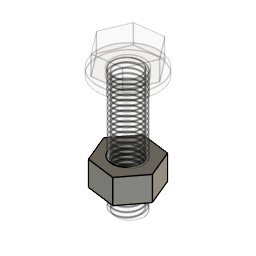
M10_Assembly_Final (Autodesk Fusion 360 design; units mm, degrees)
part number: 2026-04-25-14-00-48-438
part number: 2026-04-25-14-02-05-516
part number: 2026-04-25-14-04-24-538
part number: 2026-04-25-14-13-24-813
Autodesk Fusion 360 part; units mm, degrees
sketch "Sketch1" plane through (0, 0, 0) normal (0, 0, 1) x (1, 0, 0) in component "Washer"
  circle A0 centre (0, 0) radius 10
  circle A1 centre (0, 0) radius 5.25
  dimension "d1" = 20
  dimension "d2" = 10.5
  constraint coincident A0.centre A1.centre
  constraint concentric A0 A1
  measures "d1" diameter of A0
  measures "d2" diameter of A1
extrude "Extrude1" add sketch "Sketch1" along normal blind 2 makes body 1 in component "Washer"
sketch "Sketch1 (2)" plane through (0, 0, 2) normal (0, 0, 1) x (-1, 0, 0) in component "Bolt"
  circle A0 centre (0, 0) radius 5.25
  circle A1 centre (0, 0) radius 10
  line L0 (-3.5698, -8.5199) -> (5.5936, -7.3516)
  line L1 (5.5936, -7.3516) -> (9.1634, 1.1684)
  line L2 (9.1634, 1.1684) -> (3.5698, 8.5199)
  line L3 (3.5698, 8.5199) -> (-5.5936, 7.3516)
  line L4 (-5.5936, 7.3516) -> (-9.1634, -1.1684)
  line L5 (-9.1634, -1.1684) -> (-3.5698, -8.5199)
  dimension "d5" = 8
  constraint coincident A0.centre A1.centre
  measures "d5" distance of A0.centre L5
extrude "Extrude1'" add sketch "Sketch1 (2)" along normal blind 6.4 separate body contours A0 | L0 L1 L2 L3 L4 L5 makes body 2 in component "Bolt"
sketch "Sketch2" plane through (0, 0, 2) normal (0, 0, -1) x (1, 0, 0) in component "Bolt"
  line L0 (3.5698, -8.5199) -> (9.1634, -1.1684)
  line L1 (9.1634, -1.1684) -> (5.5936, 7.3516)
  line L2 (5.5936, 7.3516) -> (-3.5698, 8.5199)
  line L3 (-3.5698, 8.5199) -> (-9.1634, 1.1684)
  line L4 (-9.1634, 1.1684) -> (-5.5936, -7.3516)
  line L5 (-5.5936, -7.3516) -> (3.5698, -8.5199)
  circle A0 centre (0, 0) radius 5
  dimension "d8" = 10
  constraint coincident A0.centre origin
  measures "d8" diameter of A0
extrude "Extrude2" add sketch "Sketch2" along normal blind 40 contours A0 bodies 2 in component "Bolt"
thread "Thread1" "ISO Metric profile 10.0 M10x1.5 M10x1.5 6g" major diameter 9.85 minor diameter 8.141 pitch 1.5 angle 60 modelled right hand crest width 0.2177 on face at (4.9938, 0.2492, -24.6667) crest through (4.925, 0, 2.375) on bodies 2 in component "Bolt"
sketch "Sketch1 (3)" plane through (0, 0, -38) normal (0, 0, -1) x (1, 0, 0) in component "Nut"
  spline S0 degree 3 poles (-4.0519, -0.3884) (-4.055, -0.9258) (-3.9512, -1.4584) (-3.5409, -2.4749) (-3.2312, -2.9459) (-2.4367, -3.7605) (-1.9541, -4.0907) (-0.8716, -4.5594) (-0.2791, -4.6862) (0.7385, -4.7058) (1.1549, -4.6582) (1.9739, -4.4542) (2.3723, -4.2963) (2.7453, -4.0889) knots 0 0 0 0 0.161221 0.161221 0.328565 0.328565 0.502029 0.502029 0.68161 0.68161 0.806401 0.806401 0.933976 0.933976 0.933976 0.933976
  arc A0 (2.7453, -4.0889) -> (4.9137, -0.3331) centre (0, 0) ccw
  spline S1 degree 3 poles (4.9137, -0.3331) (4.9036, 0.2959) (4.7727, 0.9169) (4.2847, 2.0534) (3.9396, 2.5608) (3.0865, 3.3975) (2.5922, 3.7244) (1.5238, 4.1587) (0.9631, 4.2693) (0.0275, 4.2662) (-0.3405, 4.2169) (-1.0448, 4.0248) (-1.3786, 3.8852) (-1.6896, 3.7033) knots 0 0 0 0 0.188714 0.188714 0.371292 0.371292 0.547732 0.547732 0.718032 0.718032 0.829274 0.829274 0.937741 0.937741 0.937741 0.937741
  arc A1 (-1.6896, 3.7033) -> (-4.0519, -0.3884) centre (0, 0) ccw
  line L0 (3.5473, 8.5294) -> (-5.613, 7.3367)
  line L1 (-5.613, 7.3367) -> (-9.1603, -1.1926)
  line L2 (-9.1603, -1.1926) -> (-3.5473, -8.5294)
  line L3 (-3.5473, -8.5294) -> (5.613, -7.3367)
  line L4 (5.613, -7.3367) -> (9.1603, 1.1926)
  line L5 (9.1603, 1.1926) -> (3.5473, 8.5294)
  circle A2 centre (0, 0) radius 5
  dimension "d13" = 8
  dimension "d14" = 10
  constraint coincident A0.centre A1.centre
  measures "d13" distance of A0.centre L5
  measures "d14" diameter of A2
extrude "Extrude1''" add sketch "Sketch1 (3)" against normal blind 8 separate body contours L0 L1 L2 L3 L4 L5 makes body 3 in component "Nut"
thread "Thread1'" "ISO Metric profile 10.0 M10x1.5 M10x1.5 6H" major diameter 10.198 minor diameter 8.526 pitch 1.5 angle 60 modelled right hand crest width 0.4094 on face at (4.9752, 0.4978, -35.3333) crest through (4.263, 0, -37.625) on bodies 3 in component "Nut"
component "Washer" placed x (1, 0, 0) y (0, 1, 0) z (0, 0, 1) at (0, 0, 0)
component "Bolt" placed x (1, 0, 0) y (0, 1, 0) z (0, 0, 1) at (0, 0, 0)
component "Nut" placed x (1, 0, 0) y (0, 1, 0) z (0, 0, 1) at (0, 0, 7)
